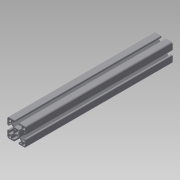
# Autodesk Inventor part: 1515-ULS
Saved by Autodesk Inventor 2013 (Build 170138000, 138)
## iProperties
Created: 2014-04-23
Part Number: 1515-ULS
Material: Generic
Document SubType Name: Modeling
Density: 1 g/cm^3
Vendor: 80/20 Inc.
Engineer: Ross Bowman
Designer: Ross Bowman
Catalog Web Link: 8020.net
Company: 80/20 Inc.
Author: Ross Bowman
Keywords: 80/20 , 8020 , T-Slot , Extrusion
Material: 6105-T5 Aluminum
Autodesk Inventor part; units mm, degrees
ref_plane "YZ Plane" through (0, 0, 0) normal (1, 0, 0) x (0, 1, 0)
ref_plane "XZ Plane" through (0, 0, 0) normal (0, 1, 0) x (-1, 0, 0)
ref_plane "XY Plane" through (0, 0, 0) normal (0, 0, 1) x (1, 0, 0)
sketch "Sketch1" plane through (0, 0, 0) normal (0, 0, 1) x (1, 0, 0)
  arc A0 (17.2516, 14.4576) -> (14.4576, 17.2516) centre (14.4576, 14.4576) ccw
  line L0 (17.2515, 12.1208) -> (17.2516, 14.4576)
  arc A1 (16.9975, 11.8668) -> (17.2515, 12.1208) centre (16.9975, 12.1208) ccw
  line L1 (12.1207, 11.8668) -> (16.9975, 11.8668)
  arc A2 (11.8667, 12.1208) -> (12.1207, 11.8668) centre (12.1207, 12.1208) ccw
  line L2 (11.8667, 16.9976) -> (11.8667, 12.1208)
  arc A3 (12.1207, 17.2516) -> (11.8667, 16.9976) centre (12.1207, 16.9976) ccw
  line L3 (14.4576, 17.2516) -> (12.1207, 17.2516)
  arc A4 (14.4576, -17.2516) -> (17.2516, -14.4576) centre (14.4576, -14.4576) ccw
  line L4 (12.1208, -17.2515) -> (14.4576, -17.2516)
  arc A5 (11.8668, -16.9975) -> (12.1208, -17.2515) centre (12.1208, -16.9975) ccw
  line L5 (11.8668, -12.1207) -> (11.8668, -16.9975)
  arc A6 (12.1208, -11.8667) -> (11.8668, -12.1207) centre (12.1208, -12.1207) ccw
  line L6 (16.9976, -11.8667) -> (12.1208, -11.8667)
  arc A7 (17.2516, -12.1207) -> (16.9976, -11.8667) centre (16.9976, -12.1207) ccw
  line L7 (17.2516, -14.4576) -> (17.2516, -12.1207)
  arc A8 (-17.2516, -14.4576) -> (-14.4576, -17.2516) centre (-14.4576, -14.4576) ccw
  line L8 (-17.2515, -12.1208) -> (-17.2516, -14.4576)
  arc A9 (-16.9975, -11.8668) -> (-17.2515, -12.1208) centre (-16.9975, -12.1208) ccw
  line L9 (-12.1207, -11.8668) -> (-16.9975, -11.8668)
  arc A10 (-11.8667, -12.1208) -> (-12.1207, -11.8668) centre (-12.1207, -12.1208) ccw
  line L10 (-11.8667, -16.9976) -> (-11.8667, -12.1208)
  arc A11 (-12.1207, -17.2516) -> (-11.8667, -16.9976) centre (-12.1207, -16.9976) ccw
  line L11 (-14.4576, -17.2516) -> (-12.1207, -17.2516)
  arc A12 (-1.178, -3.1119) -> (-1.5823, -3.1988) centre (-1.3129, -3.4682) ccw
  line L12 (-3.2921, -4.9085) -> (-1.5823, -3.1988)
  arc A13 (-3.9207, -5.1689) -> (-3.2921, -4.9085) centre (-3.9207, -4.2799) ccw
  line L13 (-4.9149, -5.1689) -> (-3.9207, -5.1689)
  arc A14 (-5.1689, -4.9149) -> (-4.9149, -5.1689) centre (-4.9149, -4.9149) ccw
  line L14 (-5.1689, -3.9207) -> (-5.1689, -4.9149)
  arc A15 (-4.9085, -3.2921) -> (-5.1689, -3.9207) centre (-4.2799, -3.9207) ccw
  line L15 (-3.1988, -1.5823) -> (-4.9085, -3.2921)
  arc A16 (-3.1988, -1.5823) -> (-3.1119, -1.178) centre (-3.4682, -1.3129) ccw
  arc A17 (-3.1119, 1.178) -> (-3.1119, -1.178) centre (0, 0) ccw
  arc A18 (-3.1119, 1.178) -> (-3.1988, 1.5823) centre (-3.4682, 1.3129) ccw
  line L16 (-4.9085, 3.2921) -> (-3.1988, 1.5823)
  arc A19 (-5.1689, 3.9207) -> (-4.9085, 3.2921) centre (-4.2799, 3.9207) ccw
  line L17 (-5.1689, 4.9149) -> (-5.1689, 3.9207)
  arc A20 (-4.9149, 5.1689) -> (-5.1689, 4.9149) centre (-4.9149, 4.9149) ccw
  line L18 (-3.9207, 5.1689) -> (-4.9149, 5.1689)
  arc A21 (-3.2921, 4.9085) -> (-3.9207, 5.1689) centre (-3.9207, 4.2799) ccw
  line L19 (-1.5823, 3.1988) -> (-3.2921, 4.9085)
  arc A22 (-1.5823, 3.1988) -> (-1.178, 3.1119) centre (-1.3129, 3.4682) ccw
  arc A23 (1.178, 3.1119) -> (-1.178, 3.1119) centre (0, 0) ccw
  arc A24 (1.178, 3.1119) -> (1.5823, 3.1988) centre (1.3129, 3.4682) ccw
  line L20 (3.2921, 4.9085) -> (1.5823, 3.1988)
  arc A25 (3.9207, 5.1689) -> (3.2921, 4.9085) centre (3.9207, 4.2799) ccw
  line L21 (4.9149, 5.1689) -> (3.9207, 5.1689)
  arc A26 (5.1689, 4.9149) -> (4.9149, 5.1689) centre (4.9149, 4.9149) ccw
  line L22 (5.1689, 3.9207) -> (5.1689, 4.9149)
  arc A27 (4.9085, 3.2921) -> (5.1689, 3.9207) centre (4.2799, 3.9207) ccw
  line L23 (3.1988, 1.5823) -> (4.9085, 3.2921)
  arc A28 (3.1988, 1.5823) -> (3.1119, 1.178) centre (3.4682, 1.3129) ccw
  arc A29 (3.1119, -1.178) -> (3.1119, 1.178) centre (0, 0) ccw
  arc A30 (3.1119, -1.178) -> (3.1988, -1.5823) centre (3.4682, -1.3129) ccw
  line L24 (4.9085, -3.2921) -> (3.1988, -1.5823)
  arc A31 (5.1689, -3.9207) -> (4.9085, -3.2921) centre (4.2799, -3.9207) ccw
  line L25 (5.1689, -4.9149) -> (5.1689, -3.9207)
  arc A32 (4.9149, -5.1689) -> (5.1689, -4.9149) centre (4.9149, -4.9149) ccw
  line L26 (3.9207, -5.1689) -> (4.9149, -5.1689)
  arc A33 (3.2921, -4.9085) -> (3.9207, -5.1689) centre (3.9207, -4.2799) ccw
  line L27 (1.5823, -3.1988) -> (3.2921, -4.9085)
  arc A34 (1.5823, -3.1988) -> (1.178, -3.1119) centre (1.3129, -3.4682) ccw
  arc A35 (-1.178, -3.1119) -> (1.178, -3.1119) centre (0, 0) ccw
  arc A36 (-14.4576, 17.2516) -> (-17.2516, 14.4576) centre (-14.4576, 14.4576) ccw
  line L28 (-12.1208, 17.2515) -> (-14.4576, 17.2516)
  arc A37 (-11.8668, 16.9975) -> (-12.1208, 17.2515) centre (-12.1208, 16.9975) ccw
  line L29 (-11.8668, 12.1207) -> (-11.8668, 16.9975)
  arc A38 (-12.1208, 11.8667) -> (-11.8668, 12.1207) centre (-12.1208, 12.1207) ccw
  line L30 (-16.9976, 11.8667) -> (-12.1208, 11.8667)
  arc A39 (-17.2516, 12.1207) -> (-16.9976, 11.8667) centre (-16.9976, 12.1207) ccw
  line L31 (-17.2516, 14.4576) -> (-17.2516, 12.1207)
  arc A40 (19.05, -5.6526) -> (17.4752, -4.0778) centre (17.4752, -5.6526) ccw
  line L32 (17.4752, -4.0778) -> (16.5608, -4.0778)
  arc A41 (16.5608, -4.0778) -> (14.986, -5.6526) centre (16.5608, -5.6526) ccw
  line L33 (14.986, -5.6526) -> (14.986, -6.6315)
  arc A42 (14.986, -6.6315) -> (15.24, -6.8855) centre (15.24, -6.6315) ccw
  line L34 (15.24, -6.8855) -> (16.5862, -6.8855)
  arc A43 (16.8402, -7.1395) -> (16.5862, -6.8855) centre (16.5862, -7.1395) ccw
  line L35 (16.8402, -7.1395) -> (16.8402, -9.4255)
  arc A44 (15.9513, -10.3145) -> (16.8402, -9.4255) centre (15.9512, -9.4255) ccw
  line L36 (15.9513, -10.3145) -> (12.38, -10.3146)
  arc A45 (11.481, -9.9417) -> (12.38, -10.3146) centre (12.38, -9.0446) ccw
  line L37 (11.481, -9.9417) -> (7.1147, -5.5659)
  arc A46 (6.7437, -4.6689) -> (7.1147, -5.5659) centre (8.0137, -4.6689) ccw
  line L38 (6.7437, -4.6689) -> (6.7437, 4.6414)
  arc A47 (7.1167, 5.5404) -> (6.7437, 4.6414) centre (8.0137, 4.6414) ccw
  line L39 (7.1167, 5.5404) -> (11.5019, 9.9161)
  arc A48 (12.399, 10.2871) -> (11.5019, 9.9161) centre (12.399, 9.0171) ccw
  line L40 (12.399, 10.2871) -> (15.9513, 10.287)
  arc A49 (16.8402, 9.398) -> (15.9513, 10.287) centre (15.9512, 9.398) ccw
  line L41 (16.8402, 9.398) -> (16.8402, 7.112)
  arc A50 (16.5862, 6.858) -> (16.8402, 7.112) centre (16.5862, 7.112) ccw
  line L42 (16.5862, 6.858) -> (15.24, 6.858)
  arc A51 (15.24, 6.858) -> (14.986, 6.604) centre (15.24, 6.604) ccw
  line L43 (14.986, 6.604) -> (14.986, 5.625)
  arc A52 (14.986, 5.625) -> (16.5608, 4.0502) centre (16.5608, 5.625) ccw
  line L44 (16.5608, 4.0502) -> (17.4752, 4.0502)
  arc A53 (17.4752, 4.0502) -> (19.05, 5.625) centre (17.4752, 5.625) ccw
  line L45 (19.05, 5.625) -> (19.05, 15.875)
  arc A54 (19.05, 15.875) -> (15.8746, 19.05) centre (15.875, 15.875) ccw
  line L46 (15.8746, 19.05) -> (5.6526, 19.05)
  arc A55 (5.6526, 19.05) -> (4.0778, 17.4752) centre (5.6526, 17.4752) ccw
  line L47 (4.0778, 17.4752) -> (4.0778, 16.5608)
  arc A56 (4.0778, 16.5608) -> (5.6526, 14.986) centre (5.6526, 16.5608) ccw
  line L48 (5.6526, 14.986) -> (6.6315, 14.986)
  arc A57 (6.6315, 14.986) -> (6.8855, 15.24) centre (6.6315, 15.24) ccw
  line L49 (6.8855, 15.24) -> (6.8855, 16.5862)
  arc A58 (7.1395, 16.8402) -> (6.8855, 16.5862) centre (7.1395, 16.5862) ccw
  line L50 (7.1395, 16.8402) -> (9.4255, 16.8402)
  arc A59 (10.3145, 15.9513) -> (9.4255, 16.8402) centre (9.4255, 15.9512) ccw
  line L51 (10.3145, 15.9513) -> (10.3146, 12.38)
  arc A60 (9.9417, 11.481) -> (10.3146, 12.38) centre (9.0446, 12.38) ccw
  line L52 (9.9417, 11.481) -> (5.5659, 7.1147)
  arc A61 (4.6689, 6.7437) -> (5.5659, 7.1147) centre (4.6689, 8.0137) ccw
  line L53 (4.6689, 6.7437) -> (-4.6414, 6.7437)
  arc A62 (-5.5404, 7.1167) -> (-4.6414, 6.7437) centre (-4.6414, 8.0137) ccw
  line L54 (-5.5404, 7.1167) -> (-9.9161, 11.5019)
  arc A63 (-10.2871, 12.399) -> (-9.9161, 11.5019) centre (-9.0171, 12.399) ccw
  line L55 (-10.2871, 12.399) -> (-10.287, 15.9513)
  arc A64 (-9.398, 16.8402) -> (-10.287, 15.9513) centre (-9.398, 15.9512) ccw
  line L56 (-9.398, 16.8402) -> (-7.112, 16.8402)
  arc A65 (-6.858, 16.5862) -> (-7.112, 16.8402) centre (-7.112, 16.5862) ccw
  line L57 (-6.858, 16.5862) -> (-6.858, 15.24)
  arc A66 (-6.858, 15.24) -> (-6.604, 14.986) centre (-6.604, 15.24) ccw
  line L58 (-6.604, 14.986) -> (-5.625, 14.986)
  arc A67 (-5.625, 14.986) -> (-4.0502, 16.5608) centre (-5.625, 16.5608) ccw
  line L59 (-4.0502, 16.5608) -> (-4.0502, 17.4752)
  arc A68 (-4.0502, 17.4752) -> (-5.625, 19.05) centre (-5.625, 17.4752) ccw
  line L60 (-5.625, 19.05) -> (-15.875, 19.05)
  arc A69 (-15.875, 19.05) -> (-19.05, 15.8746) centre (-15.875, 15.875) ccw
  line L61 (-19.05, 15.8746) -> (-19.05, 5.6526)
  arc A70 (-19.05, 5.6526) -> (-17.4752, 4.0778) centre (-17.4752, 5.6526) ccw
  line L62 (-17.4752, 4.0778) -> (-16.5608, 4.0778)
  arc A71 (-16.5608, 4.0778) -> (-14.986, 5.6526) centre (-16.5608, 5.6526) ccw
  line L63 (-14.986, 5.6526) -> (-14.986, 6.6315)
  arc A72 (-14.986, 6.6315) -> (-15.24, 6.8855) centre (-15.24, 6.6315) ccw
  line L64 (-15.24, 6.8855) -> (-16.5862, 6.8855)
  arc A73 (-16.8402, 7.1395) -> (-16.5862, 6.8855) centre (-16.5862, 7.1395) ccw
  line L65 (-16.8402, 7.1395) -> (-16.8402, 9.4255)
  arc A74 (-15.9513, 10.3145) -> (-16.8402, 9.4255) centre (-15.9512, 9.4255) ccw
  line L66 (-15.9513, 10.3145) -> (-12.38, 10.3146)
  arc A75 (-11.481, 9.9417) -> (-12.38, 10.3146) centre (-12.38, 9.0446) ccw
  line L67 (-11.481, 9.9417) -> (-7.1147, 5.5659)
  arc A76 (-6.7437, 4.6689) -> (-7.1147, 5.5659) centre (-8.0137, 4.6689) ccw
  line L68 (-6.7437, 4.6689) -> (-6.7437, -4.6414)
  arc A77 (-7.1167, -5.5404) -> (-6.7437, -4.6414) centre (-8.0137, -4.6414) ccw
  line L69 (-7.1167, -5.5404) -> (-11.5019, -9.9161)
  arc A78 (-12.399, -10.2871) -> (-11.5019, -9.9161) centre (-12.399, -9.0171) ccw
  line L70 (-12.399, -10.2871) -> (-15.9513, -10.287)
  arc A79 (-16.8402, -9.398) -> (-15.9513, -10.287) centre (-15.9512, -9.398) ccw
  line L71 (-16.8402, -9.398) -> (-16.8402, -7.112)
  arc A80 (-16.5862, -6.858) -> (-16.8402, -7.112) centre (-16.5862, -7.112) ccw
  line L72 (-16.5862, -6.858) -> (-15.24, -6.858)
  arc A81 (-15.24, -6.858) -> (-14.986, -6.604) centre (-15.24, -6.604) ccw
  line L73 (-14.986, -6.604) -> (-14.986, -5.625)
  arc A82 (-14.986, -5.625) -> (-16.5608, -4.0502) centre (-16.5608, -5.625) ccw
  line L74 (-16.5608, -4.0502) -> (-17.4752, -4.0502)
  arc A83 (-17.4752, -4.0502) -> (-19.05, -5.625) centre (-17.4752, -5.625) ccw
  line L75 (-19.05, -5.625) -> (-19.05, -15.875)
  arc A84 (-19.05, -15.875) -> (-15.8746, -19.05) centre (-15.875, -15.875) ccw
  line L76 (-15.8746, -19.05) -> (-5.6526, -19.05)
  arc A85 (-5.6526, -19.05) -> (-4.0778, -17.4752) centre (-5.6526, -17.4752) ccw
  line L77 (-4.0778, -17.4752) -> (-4.0778, -16.5608)
  arc A86 (-4.0778, -16.5608) -> (-5.6526, -14.986) centre (-5.6526, -16.5608) ccw
  line L78 (-5.6526, -14.986) -> (-6.6315, -14.986)
  arc A87 (-6.6315, -14.986) -> (-6.8855, -15.24) centre (-6.6315, -15.24) ccw
  line L79 (-6.8855, -15.24) -> (-6.8855, -16.5862)
  arc A88 (-7.1395, -16.8402) -> (-6.8855, -16.5862) centre (-7.1395, -16.5862) ccw
  line L80 (-7.1395, -16.8402) -> (-9.4255, -16.8402)
  arc A89 (-10.3145, -15.9513) -> (-9.4255, -16.8402) centre (-9.4255, -15.9512) ccw
  line L81 (-10.3145, -15.9513) -> (-10.3146, -12.38)
  arc A90 (-9.9417, -11.481) -> (-10.3146, -12.38) centre (-9.0446, -12.38) ccw
  line L82 (-9.9417, -11.481) -> (-5.5659, -7.1147)
  arc A91 (-4.6689, -6.7437) -> (-5.5659, -7.1147) centre (-4.6689, -8.0137) ccw
  line L83 (-4.6689, -6.7437) -> (4.6414, -6.7437)
  arc A92 (5.5404, -7.1167) -> (4.6414, -6.7437) centre (4.6414, -8.0137) ccw
  line L84 (5.5404, -7.1167) -> (9.9161, -11.5019)
  arc A93 (10.2871, -12.399) -> (9.9161, -11.5019) centre (9.0171, -12.399) ccw
  line L85 (10.2871, -12.399) -> (10.287, -15.9513)
  arc A94 (9.398, -16.8402) -> (10.287, -15.9513) centre (9.398, -15.9512) ccw
  line L86 (9.398, -16.8402) -> (7.112, -16.8402)
  arc A95 (6.858, -16.5862) -> (7.112, -16.8402) centre (7.112, -16.5862) ccw
  line L87 (6.858, -16.5862) -> (6.858, -15.24)
  arc A96 (6.858, -15.24) -> (6.604, -14.986) centre (6.604, -15.24) ccw
  line L88 (6.604, -14.986) -> (5.625, -14.986)
  arc A97 (5.625, -14.986) -> (4.0502, -16.5608) centre (5.625, -16.5608) ccw
  line L89 (4.0502, -16.5608) -> (4.0502, -17.4752)
  arc A98 (4.0502, -17.4752) -> (5.625, -19.05) centre (5.625, -17.4752) ccw
  line L90 (5.625, -19.05) -> (15.875, -19.05)
  arc A99 (15.875, -19.05) -> (19.05, -15.8746) centre (15.875, -15.875) ccw
  line L91 (19.05, -15.8746) -> (19.05, -5.6526)
  constraints: 200 point on circle, 184 end point, 100 centre point
extrude "Extrusion1" add sketch "Sketch1" against normal blind 304.8
body "Solid1"
